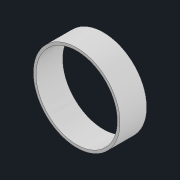
# Autodesk Inventor part: A6063-PP-65-2-30
Saved by Autodesk Inventor 2022 (Build 260153000, 153)
## iProperties
Created: 2024-06-02
Part Number: A6063-PP-65-2-30
Material: 一般
Document SubType Name: Modeling
Designer: gisen
Density: 1 g/cm^3
Appearance: 既定
Author: gisen
Autodesk Inventor part; units mm, degrees
ref_plane "YZ Plane" through (0, 0, 0) normal (1, 0, 0) x (0, 1, 0)
ref_plane "XZ Plane" through (0, 0, 0) normal (0, 1, 0) x (-1, 0, 0)
ref_plane "XY Plane" through (0, 0, 0) normal (0, 0, 1) x (1, 0, 0)
sketch "スケッチ1" plane through (0, 0, 0) normal (0, 0, 1) x (1, 0, 0)
  circle A0 centre (0, 0) radius 30.5
  circle A1 centre (0, 0) radius 32.5
  dimension "d0" = 61
  dimension "d1" = 65
  constraints: 2 centre point, 2 coincident
  measures "d0" diameter of A0
  measures "d1" diameter of A1
extrude "押し出し1" add sketch "スケッチ1" along normal mid plane 20
